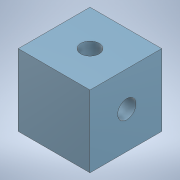
# Autodesk Inventor part: AxisConnector
Saved by Autodesk Inventor 2022 (Build 260153000, 153)
## iProperties
Created: 2021-04-24
Part Number: AxisConnector
Material: Generic
Document SubType Name: Modeling
Designer: Mick Veldhuis
Density: 1 g/cm^3
Appearance: Default
Author: Mick Veldhuis
Autodesk Inventor part; units mm, degrees
ref_plane "YZ Plane" through (0, 0, 0) normal (1, 0, 0) x (0, 1, 0)
ref_plane "XZ Plane" through (0, 0, 0) normal (0, 1, 0) x (-1, 0, 0)
ref_plane "XY Plane" through (0, 0, 0) normal (0, 0, 1) x (1, 0, 0)
sketch "Sketch1" plane through (0, 0, 0) normal (0, 1, 0) x (-1, 0, 0)
  line L0 (-78, 78) -> (78, 78)
  line L1 (78, 78) -> (78, -78)
  line L2 (78, -78) -> (-78, -78)
  line L3 (-78, -78) -> (-78, 78)
  line L4 (-78, 78) -> (78, -78) construction
  line L5 (78, 78) -> (-78, -78) construction
  point P0 (0, 0)
  dimension "d0" = 156
  dimension "d1" = 156
  constraints: 12 end point, 2 midpoint, 2 parallel, 1 horizontal, 1 perpendicular
  measures "d0" distance of L1.end L2.end
  measures "d1" distance of L0.end L1.end
extrude "Body" add sketch "Sketch1" along normal blind 156
sketch "Sketch2" plane through (78, 0, 78) normal (1, 0, 0) x (0, 0, -1)
  circle A0 centre (80, 80) radius 20
  point P0 (78, 0)
  constraints: 1 centre point
extrude "RotAxis" cut sketch "Sketch2" against normal through all
sketch "Sketch4" plane through (0, 156, 0) normal (0, 1, 0) x (1, 0, 0)
  circle A0 centre (0, 0) radius 20
  constraints: 1 centre point, 1 coincident
extrude "CableHole" cut sketch "Sketch4" against normal through all
sketch "Sketch5" plane through (0, 0, 0) normal (0, -1, 0) x (1, 0, 0)
  point P0 (0, 0)
  point P1 (-58, 58)
  point P2 (-58, -58)
  point P3 (58, -58)
  point P4 (58, 58)
hole "BoltHoles" at (-58, 0, 58) at (-58, 0, -58) at (58, 0, -58) at (58, 0, 58) direction (0, 1, 0) diameter 6 depth 20 tip angle 118
body "Solid1"
